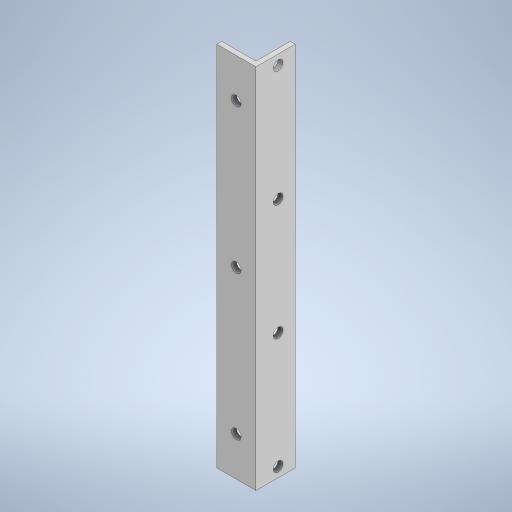
# Autodesk Inventor part: Cylinder Bracket
Saved by Autodesk Inventor 2023 (Build 270158000, 158)
## iProperties
Created: 2022-10-26
Part Number: Cylinder Bracket
Material: Generic
Document SubType Name: Modeling
Designer: tommy
Density: 1 g/cm^3
Appearance: Default
Author: tommy
Autodesk Inventor part; units mm, degrees
ref_plane "YZ Plane" through (0, 0, 0) normal (1, 0, 0) x (0, 1, 0)
ref_plane "XZ Plane" through (0, 0, 0) normal (0, 1, 0) x (-1, 0, 0)
ref_plane "XY Plane" through (0, 0, 0) normal (0, 0, 1) x (1, 0, 0)
sketch "Sketch1" plane through (0, 0, 0) normal (0, 1, 0) x (-1, 0, 0)
  line L0 (0, 0) -> (0, -25.4)
  line L1 (0, -25.4) -> (3.175, -25.4)
  line L2 (3.175, -25.4) -> (3.175, -3.175)
  line L3 (3.175, -3.175) -> (25.4, -3.175)
  line L4 (25.4, -3.175) -> (25.4, 0)
  line L5 (25.4, 0) -> (0, 0)
  dimension "d0" = 25.4
  dimension "d1" = 3.175
  dimension "d2" = 22.225
  dimension "d3" = 22.225
  constraints: 12 end point, 5 perpendicular, 1 vertical
  measures "d0" distance of L0.start L0.end
  measures "d1" distance of L0.end L1.end
  measures "d2" distance of L1.end L2.end
  measures "d3" distance of L2.end L3.end
extrude "Extrusion1" add sketch "Sketch1" along normal blind 237.49
sketch "Sketch4" plane through (0, 0, 0) normal (1, 0, 0) x (0, 0, -1)
  line L0 (25.4, 0) -> (3.175, 0) projected
  line L1 (25.4, 237.49) -> (3.175, 237.49) projected
  circle A0 centre (14.2875, 231.14) radius 3.175
  circle A1 centre (14.2875, 6.35) radius 3.175
  circle A2 centre (14.2875, 156.21) radius 3.175
  circle A3 centre (14.2875, 81.28) radius 3.175
  point P0 (0, 0)
  dimension "d23" = 6.35
  dimension "d26" = 6.35
  dimension "d27" = 6.35
  constraints: 4 centre point
  measures "d23" diameter of A1
  measures "d26" diameter of A2
  measures "d27" diameter of A3
extrude "Extrusion4" cut sketch "Sketch4" against normal blind 237.49
sketch "Sketch5" plane through (-25.4, 0, 0) normal (0, 0, 1) x (1, 0, 0)
  line L0 (0, 0) -> (25.4, 0) projected
  line L1 (22.225, 237.49) -> (0, 237.49) projected
  circle A0 centre (12.7, 212.09) radius 3.175
  circle A1 centre (12.7, 118.745) radius 3.175
  circle A2 centre (12.7, 25.4) radius 3.175
  dimension "d32" = 6.35
  dimension "d33" = 6.35
  dimension "d34" = 6.35
  constraints: 3 centre point
  measures "d32" diameter of A0
  measures "d33" diameter of A1
  measures "d34" diameter of A2
extrude "Extrusion5" cut sketch "Sketch5" against normal blind 237.49
body "Solid1"
